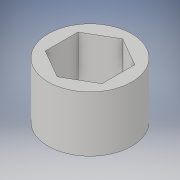
# Autodesk Inventor part: ShaftSpacer0.5inHex
Saved by Autodesk Inventor 2018 (Build 220112000, 112)
## iProperties
Created: 2019-09-28
Part Number: ShaftSpacer0.5inHex
Material: Generic
Document SubType Name: Modeling
Designer: snipe
Density: 1 g/cm^3
Appearance: Default
Author: snipe
Autodesk Inventor part; units mm, degrees
ref_plane "YZ Plane" through (0, 0, 0) normal (1, 0, 0) x (0, 1, 0)
ref_plane "XZ Plane" through (0, 0, 0) normal (0, 1, 0) x (-1, 0, 0)
ref_plane "XY Plane" through (0, 0, 0) normal (0, 0, 1) x (1, 0, 0)
sketch "Sketch1" plane through (0, 0, 0) normal (0, 1, 0) x (-1, 0, 0)
  line L0 (0, -13.335) -> (0, 13.335) projected
  line L1 (-13.335, 0) -> (13.335, 0) projected
  circle A0 centre (0, 0) radius 9.525
  dimension "d0" = 19.05
  constraints: 1 centre point, 1 coincident
  measures "d0" diameter of A0
extrude "Extrusion1" add sketch "Sketch1" along normal blind 12.7
sketch "Sketch2" plane through (0, 12.7, 0) normal (0, 1, 0) x (1, 0, 0)
  line L0 (0, 7.479) -> (6.477, 3.7395)
  line L1 (6.477, 3.7395) -> (6.477, -3.7395)
  line L2 (6.477, -3.7395) -> (0, -7.479)
  line L3 (0, -7.479) -> (-6.477, -3.7395)
  line L4 (-6.477, -3.7395) -> (-6.477, 3.7395)
  line L5 (-6.477, 3.7395) -> (0, 7.479)
  point P0 (0, 0)
  point P1 (0, 0)
  dimension "d3" = 12.954
  constraints: 12 end point, 1 coincident, 13 other
  measures "d3" distance between parallel lines of L1 L4
extrude "Extrusion2" cut sketch "Sketch2" against normal through all
body "Solid1"
